1 element test fit 1 4_v11 (Autodesk Fusion 360 design; units mm, degrees)
Autodesk Fusion 360 part; units mm, degrees
note: some values were not read from the file. Chosen so that the rebuilt part matches the saved one: which face or edge a step refers to. Set by a fixed rule: which sketch regions a step uses.
sketch "Box All Sketch" plane through (0, 0, 0) normal (0, 0, 1) x (1, 0, 0)
  line L0 (0, 0) -> (-160, 0)
  line L1 (-160, 0) -> (-160, 9)
  line L2 (-160, 9) -> (0, 9)
  line L3 (0, 9) -> (0, 0)
  line L4 (-160, 0) -> (-144.925, 0)
  line L5 (-144.925, 0) -> (-144.925, 3.175)
  line L6 (-144.925, 3.175) -> (-135.075, 3.175)
  line L7 (-135.075, 3.175) -> (-135.075, 0)
  circle A0 centre (-144.5047, 2.6047) radius 0.7005
  circle A1 centre (-135.4953, 2.6047) radius 0.7005
  circle A2 centre (-302, 114) radius 1.05
  circle A3 centre (-154, 222) radius 1.05
  circle A4 centre (-302, 222) radius 1.05
  line L8 (-84.9035, 14.983) -> (-82.8935, 14.983)
  line L9 (-82.8935, 14.983) -> (-82.8935, -14.3686)
  line L10 (-82.8935, -14.3686) -> (-84.9035, -14.3686)
  line L11 (-84.9035, -14.3686) -> (-84.9035, 14.983)
  line L12 (-82.8935, 14.983) -> (-82.8935, -14.3686)
  line L13 (-84.9035, -14.3686) -> (-84.9035, 14.983)
  line L14 (-160, 16.9345) -> (-135.3509, 16.9345)
  line L15 (-135.3509, 16.9345) -> (-135.3509, -20.7163)
  line L16 (-135.3509, -20.7163) -> (-160, -20.7163)
  line L17 (-160, -20.7163) -> (-160, 16.9345)
  line L18 (-29.0515, 14.2128) -> (0.4341, 14.2128)
  line L19 (0.4341, 14.2128) -> (0.4341, -10.7366)
  line L20 (0.4341, -10.7366) -> (-29.0515, -10.7366)
  line L21 (-29.0515, -10.7366) -> (-29.0515, 14.2128)
  dimension "d8" = 9
  dimension "d12" = 9.85
  dimension "d13" = 3.175
  dimension "d14" = 3.175
  dimension "d34" = 1.401
  dimension "d36" = 0.4203
  dimension "d37" = 0.5703
  dimension "d38" = 0.4203
  dimension "d177" = 160
  dimension "d189" = 15.075
  dimension "d480" = 2.01
  dimension "d483" = 2.01
  dimension "d484" = 24.6491
  dimension "d485" = 37.6508
  dimension "d486" = 29.4856
  dimension "d487" = 24.9494
  constraint horizontal L0
  constraint vertical L1
  constraint horizontal L2
  constraint vertical L3
  constraint coincident L0.start L3.end
  constraint horizontal L4
  constraint perpendicular L4 L5
  constraint perpendicular L5 L6
  constraint perpendicular L6 L7
  constraint equal A0 A1
  constraint horizontal A0.centre A1.centre
  constraint horizontal L8
  constraint vertical L9
  constraint horizontal L10
  constraint vertical L11
  constraint vertical L12
  constraint vertical L13
  constraint horizontal L14
  constraint vertical L15
  constraint horizontal L16
  constraint vertical L17
  constraint horizontal L18
  constraint vertical L19
  constraint horizontal L20
  constraint vertical L21
  measures "d8" distance of L0.start L2.end
  measures "d12" distance of L5.end L6.end
  measures "d13" distance of L4.end L5.end
  measures "d14" distance of L6.end L7.end
  measures "d34" diameter of A0
  measures "d36" distance of L5 A0.centre
  measures "d37" distance of L6 A0.centre
  measures "d38" horizontal distance of L7.end A1.centre
  measures "d177" distance of L1 L3
  measures "d189" distance of L1 L5
  measures "d480" distance of L8.start L8.end
  measures "d483" distance of L8.start L8.end
  measures "d484" distance of L14.start L14.end
  measures "d485" distance of L14.start L16.end
  measures "d486" distance of L18.start L18.end
  measures "d487" distance of L18.start L20.end
extrude "Extrude Box Bottom and Top" add sketch "Box All Sketch" along normal blind 3.175 contours L0 L1 L2 L4 L5 L6 A0 A1 L15 L17 | L0 L2 L6 L7 A1 L11 L13 L15 | L0 L2 L9 L11 L12 L13 | L0 L2 L9 L12 L21 | L0 L2 L3 L21 makes body 1
pattern_linear "bottom length repeat holes" count 7 spacing 20 along (1, 0, 0) of 13 faces at (-144.925, 0.6814, 1.0583) (-144.925, 3.1684, 1.0583) (-145.103, 2.9689, 2.1167) (-144.4245, 3.3006, 2.1167) (-144.9205, 3.175, 1.0583) (-141.366, 3.175, 1.0583) (-135.0841, 3.175, 1.0583) (-135.6069, 3.2962, 2.1167) (-135.2285, 3.2524, 2.1167) (-134.8758, 2.9317, 2.1167) (-134.862, 2.3053, 2.1167) (-135.075, 3.1717, 1.0583) (-135.075, 1.3629, 1.0583) on bodies 1
extrude "Extrude20" cut sketch "Box All Sketch" along normal blind 3.175 contours L0 L1 L2 L4 L5 L6 A0 A1 L15 L17 | L0 L2 L9 L11 L12 L13 | L0 L2 L3 L21 bodies 1 makes body 2 at (-55.8135, 7.1017, 0)
equation "fingerWidth = 10 mm"
equation "length = 160 mm"
equation "thickness = 3.175 mm"
equation "height = 50 mm"
equation "d12 = holeWidth"
equation "d13 = thickness"
equation "d14 = thickness"
equation "d15 = thickness"
equation "d21 = lengthCutsBottom"
equation "d23 = -2 * fingerWidth"
equation "toolDiameter = 1.401 mm"
equation "d34 = toolDiameter"
equation "d36 = boneCornerToCenterSide"
equation "d37 = boneCornerToCenter"
equation "d38 = boneCornerToCenterSide"
equation "boneCornerToCenter = toolDiameter / 2 / sqrt(2) - 1 * kerf" comment "Best: 2.001 -2*kerf, 0.1;;;Best: 2.001 no kerf and 0.1   OLD+6 kerf at 2.001 Diam and .1 mm"
equation "tempLengthPiecesBottom = ceil(( ( floor(( length - 2 * thickness ) / fingerWidth) - 2 ) - ( ( floor(( length - 2 * thickness ) / fingerWidth) - 2 ) % 2 - 1 ) ))"
equation "lengthCutsBottom = ceil(tempLengthPiecesBottom / 2)"
equation "lengthShoulder = ( length - fingerWidth * tempLengthPiecesBottom ) / 2 - kerf"
equation "depth = 120 mm"
equation "tempDepthPiecesBottom = ceil(( ( floor(( depth - 2 * thickness ) / fingerWidth) - 2 ) - ( ( floor(( depth - 2 * thickness ) / fingerWidth) - 2 ) % 2 - 1 ) ))"
equation "depthCutsSideBottom = ceil(tempDepthPiecesBottom / 2)"
equation "depthShoulder = ( depth - fingerWidth * tempDepthPiecesBottom ) / 2 - kerf"
equation "tempHeightPiecesSide = ceil(( ( floor(( height - 2 * thickness ) / fingerWidth) - 2 ) - ( ( floor(( height - 2 * thickness ) / fingerWidth) - 2 ) % 2 - 1 ) ))"
equation "heightCutsSide = ceil(tempHeightPiecesSide / 2)"
equation "heightSholder = ( height - fingerWidth * tempHeightPiecesSide ) / 2 - kerf"
equation "d177 = length"
equation "d189 = lengthShoulder"
equation "kerf = -0.075 mm"
equation "holeWidth = fingerWidth + 2 * kerf"
equation "lengthShoulderHole = lengthShoulder + 2 * kerf"
equation "depthShouderHole = depthShoulder + 2 * kerf"
equation "heightShoulderHole = heightSholder + 2 * kerf"
equation "assembleScrewDiam = 2.1 mm"
equation "assembleScrewDistance = 6 mm"
equation "assembleAvoidCollisionDistance = 1 mm"
equation "coolingHoleDistance = 8 mm"
equation "boneCornerToCenterPack = -2 * kerf"
equation "boneCornerToCenterSide = boneCornerToCenter - boneCornerToCenterPack"
